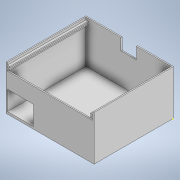
# Autodesk Inventor part: casingN
Saved by Autodesk Inventor 2022 (Build 260153000, 153)
## iProperties
Created: 2023-02-13
Part Number: casingN
Material: Generic
Document SubType Name: Modeling
Designer: biom
Density: 1 g/cm^3
Appearance: Default
Author: biom
Autodesk Inventor part; units mm, degrees
ref_plane "YZ Plane" through (0, 0, 0) normal (1, 0, 0) x (0, 1, 0)
ref_plane "XZ Plane" through (0, 0, 0) normal (0, 1, 0) x (-1, 0, 0)
ref_plane "XY Plane" through (0, 0, 0) normal (0, 0, 1) x (1, 0, 0)
sketch "Sketch1" plane through (0, 0, 0) normal (0, 1, 0) x (-1, 0, 0)
  line L0 (0, 0) -> (113.5, 0)
  line L1 (113.5, 0) -> (113.5, -103)
  line L2 (113.5, -103) -> (0, -103)
  line L3 (0, -103) -> (0, 0)
  dimension "d0" = 113.5
  dimension "d1" = 103
  constraints: 8 end point, 2 parallel, 1 horizontal, 1 perpendicular
  measures "d0" distance of L1.end L2.end
  measures "d1" distance of L0.end L1.end
extrude "Extrusion1" add sketch "Sketch1" along normal blind 3
sketch "Sketch2" plane through (0, 3, 0) normal (0, 1, 0) x (1, 0, 0)
  line L0 (0, 0) -> (0, 103) projected
  line L1 (-113.5, 0) -> (0, 0) projected
  line L2 (0, 103) -> (-113.5, 103) projected
  line L3 (-113.5, 103) -> (-113.5, 0) projected
  line L4 (-112, 51.5) -> (-112, 0)
  line L5 (-56.75, 101.5) -> (-112, 101.5)
  line L6 (-112, 101.5) -> (-1.5, 101.5)
  line L7 (-1.5, 101.5) -> (-1.5, 0)
  line L8 (-112, 0) -> (-112, 101.5)
  constraints: 10 end point, 2 perpendicular, 2 point on line
extrude "Extrusion2" add sketch "Sketch2" along normal blind 55 contours L1 L7 L6 L5 L8 L4 L3 L2 L0
sketch "Sketch3" plane through (-112, 3, -101.5) normal (0, 0, 1) x (1, 0, 0)
  point P0 (112, -3)
sketch "Sketch4" plane through (-112, 3, -101.5) normal (0, 0, 1) x (1, 0, 0)
  line L0 (0, 55) -> (110.5, 55) projected
  line L1 (65.25, 40) -> (45.25, 40)
  line L2 (45.25, 40) -> (45.25, 55)
  line L3 (65.25, 40) -> (65.25, 55)
  line L4 (45.25, 55) -> (65.25, 55)
  point P0 (112, -3)
  dimension "d11" = 20
  constraints: 8 end point, 2 point on line, 1 collinear, 1 parallel, 1 perpendicular
  measures "d11" distance of L1.start L1.end
extrude "Extrusion3" cut sketch "Sketch4" against normal through all
sketch "Sketch5" plane through (-112, 3, 0) normal (1, 0, 0) x (0, 0, -1)
  line L0 (0, 55) -> (101.5, 55) projected
  line L1 (0, 0) -> (0, 55) projected
  line L2 (0, 52.0001) -> (101.5, 52.0001)
  line L3 (101.5, 0) -> (101.5, 55) projected
  line L4 (101.5, 52.0001) -> (101.5, 50.5001)
  line L5 (101.5, 50.5001) -> (0, 50.5001)
  line L6 (0, 52.0001) -> (0, 50.5001)
  line L7 (0, 49.0001) -> (101.5, 49.0001)
  line L8 (101.5, 49.0001) -> (101.5, 47.5001)
  line L9 (101.5, 47.5001) -> (0, 47.5001)
  line L10 (0, -3) -> (0, 55) projected
  line L11 (0, 49.0001) -> (0, 47.5001)
  dimension "d14" = 1.5
  dimension "d15" = 1.5
  dimension "d16" = 1.5
  constraints: 16 end point, 8 point on line, 3 perpendicular, 2 collinear
  measures "d14" distance of L2.end L4.end
  measures "d15" distance of L5.end L7.start
  measures "d16" distance of L7.end L8.end
extrude "Extrusion4" add sketch "Sketch5" along normal blind 3 contours L2 L3 L5 L1 | L7 L3 L9 L1
sketch "Sketch6" plane through (-1.5, 3, -101.5) normal (-1, 0, 0) x (0, 0, 1)
  line L0 (0, 55) -> (101.5, 55) projected
  line L1 (0, 0) -> (0, 55) projected
  line L2 (0, 52) -> (101.5, 52)
  line L3 (101.5, 0) -> (101.5, 55) projected
  line L4 (101.5, 52) -> (101.5, 50.5)
  line L5 (101.5, 50.5) -> (0, 50.5)
  line L6 (0, 50.5) -> (0, 52)
  line L7 (101.5, 49) -> (0, 49)
  line L8 (0, 49) -> (0, 47.5)
  line L9 (0, 47.5) -> (101.5, 47.5)
  line L10 (101.5, -3) -> (101.5, 55) projected
  line L11 (101.5, 49) -> (101.5, 47.5)
  dimension "d20" = 1.5
  dimension "d21" = 1.5
  dimension "d22" = 1.5
  constraints: 16 end point, 6 perpendicular, 6 point on line
  measures "d20" distance of L2.end L4.end
  measures "d21" distance of L4.end L7.start
  measures "d22" distance of L7.end L8.end
extrude "Extrusion5" add sketch "Sketch6" along normal blind 3 contours L2 L3 L5 L1 | L7 L3 L9 L1
sketch "Sketch8" plane through (-1.5, 3, -101.5) normal (-1, 0, 0) x (0, 0, 1)
  line L0 (101.5, 0) -> (101.5, 47.5) projected
  line L1 (101.5, 45.3848) -> (101.5, 43.8848)
  line L2 (101.5, 45.3848) -> (100, 45.3848)
  line L3 (100, 45.3848) -> (100, 24.9998)
  line L4 (100, 24.9998) -> (101.5, 24.9998)
  line L5 (101.5, -3) -> (101.5, 55) projected
  dimension "d27" = 1.5
  dimension "d28" = 1.5
  dimension "d29" = 20.385
  constraints: 8 end point, 3 point on line, 1 horizontal, 1 perpendicular, 1 vertical
  measures "d27" distance of L1.start L1.end
  measures "d28" distance of L1.start L2.end
  measures "d29" distance of L2.end L3.end
extrude "Extrusion6" add sketch "Sketch8" along normal up to surface (110.5 mm away)
sketch "Sketch10" plane through (-112, 27.9998, -1.5) normal (0, -1, 0) x (1, 0, 0)
  line L0 (110.5, 1.5) -> (0, 1.5) projected
  line L1 (33.533, 1.5) -> (33.533, 0)
  line L2 (110.5, 0) -> (0, 0) projected
  line L3 (33.4948, 1.5) -> (110.5, 1.5)
  line L4 (110.5, 1.5) -> (110.5, 0) projected
  line L5 (110.5, 1.5) -> (110.5, 0)
  line L6 (110.5, 0) -> (33.533, 0)
  point P0 (112, 1.5)
  constraints: 8 end point, 3 point on line, 2 collinear, 1 vertical
extrude "Extrusion7" add sketch "Sketch10" along normal up to surface (24.9998 mm away)
body "Solid1"
